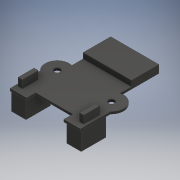
# Autodesk Inventor part: Encoder
Saved by Autodesk Inventor 2017 (Build 210142000, 142)
## iProperties
Part Number: Encoder
Material: Plástico ABS
Document SubType Name: Modeling
Designer: fam
Density: 1.06 g/cm^3
Appearance: Suave - Negro
Author: fam
Autodesk Inventor part; units mm, degrees
ref_plane "YZ Plane" through (0, 0, 0) normal (1, 0, 0) x (0, 1, 0)
ref_plane "XZ Plane" through (0, 0, 0) normal (0, 1, 0) x (-1, 0, 0)
ref_plane "XY Plane" through (0, 0, 0) normal (0, 0, 1) x (1, 0, 0)
sketch "Boceto1" plane through (0, 0, 0) normal (0, 0, 1) x (1, 0, 0)
  line L0 (-8, 26.74) -> (8, 26.74)
  line L1 (8, 26.74) -> (8, 0)
  line L2 (8, 0) -> (-8, 0)
  line L3 (-8, 0) -> (-8, 26.74)
  line L4 (6.17, 7.0485) -> (11.67, 7.0485)
  line L5 (11.67, 7.0485) -> (11.67, -3)
  line L6 (11.67, -3) -> (6.17, -3)
  line L7 (6.17, -3) -> (6.17, 7.0485)
  line L8 (-11.67, 7.0485) -> (-6.17, 7.0485)
  line L9 (-6.17, 7.0485) -> (-6.17, -3)
  line L10 (-6.17, -3) -> (-11.67, -3)
  line L11 (-11.67, -3) -> (-11.67, 7.0485)
  circle A0 centre (-9, 10) radius 1
  circle A1 centre (9, 10) radius 1
  circle A2 centre (-9, 10) radius 3.98
  circle A3 centre (9, 10) radius 3.98
  point P0 (0, 0)
  point P1 (0, 0)
  dimension "d0" = 16
  dimension "d1" = 26.74
  dimension "d2" = 5.5
  dimension "d3" = 23.34
  dimension "d6" = 11.67
  dimension "d7" = 29.74
  dimension "d8" = 2
  dimension "d9" = 25.96
  dimension "d10" = 13
  constraints: 24 end point, 6 horizontal, 6 vertical, 3 centre point, 3 horizontal alignment, 2 tangent, 1 coincident, 1 collinear, 1 concentric, 1 equal radius, 1 midpoint, 5 other
  measures "d0" distance of L1.end L2.end
  measures "d1" distance of L0.end L1.end
  measures "d2" distance of L5.end L6.end
  measures "d3" distance between parallel lines of L11 L5
  measures "d6" distance from line of point (0, 0) L5
  measures "d7" distance between parallel lines of L6 L0
  measures "d8" diameter of A1
  measures "d10" distance from line of L6 point (9, 10)
extrude "Extrusión1" add sketch "Boceto1" along normal blind 0.74
sketch "Boceto2" plane through (0, 0, 0.74) normal (0, 0, 1) x (1, 0, 0)
  line L0 (-8, 26.74) -> (8, 26.74)
  line L1 (8, 26.74) -> (8, 17.62)
  line L2 (8, 17.62) -> (-8, 17.62)
  line L3 (-8, 17.62) -> (-8, 26.74)
  point P0 (0, 0)
  dimension "d13" = 9.12
  constraints: 8 end point, 2 coincident, 2 horizontal, 2 vertical
  measures "d13" distance of L0.end L1.end
extrude "Extrusión2" add sketch "Boceto2" along normal blind 1.82
sketch "Boceto3" plane through (0, 0, 0.74) normal (0, 0, 1) x (1, 0, 0)
  line L0 (9.5, 4.2) -> (10.88, 4.2)
  line L1 (10.88, 4.2) -> (10.88, -1.1)
  line L2 (10.88, -1.1) -> (9.5, -1.1)
  line L3 (9.5, -1.1) -> (9.5, 4.2)
  line L4 (-10.88, 4.2) -> (-9.5, 4.2)
  line L5 (-9.5, 4.2) -> (-9.5, -1.1)
  line L6 (-9.5, -1.1) -> (-10.88, -1.1)
  line L7 (-10.88, -1.1) -> (-10.88, 4.2)
  line L8 (-11.67, 7.0485) -> (-11.67, -3) projected
  line L9 (6.17, -3) -> (11.67, -3) projected
  point P0 (0, 0)
  dimension "d16" = 5.3
  dimension "d17" = 1.38
  dimension "d18" = 19
  dimension "d19" = 0.79
  dimension "d20" = 7.2
  constraints: 16 end point, 4 horizontal, 3 equal length, 2 horizontal alignment, 2 vertical, 1 point on line
  measures "d16" distance of L6.end L4.start
  measures "d17" distance of L4.start L4.end
  measures "d18" distance between parallel lines of L3 L5
  measures "d19" distance between parallel lines of L8 L7
  measures "d20" distance between parallel lines of L9 L0
extrude "Extrusión3" add sketch "Boceto3" along normal blind 2.63
sketch "Boceto4" plane through (0, 0, 0) normal (0, 0, -1) x (-1, 0, 0)
  line L0 (-6.78, -2.6) -> (-11.54, -2.6)
  line L1 (-11.54, -2.6) -> (-11.54, 5.54)
  line L2 (-11.54, 5.54) -> (-6.78, 5.54)
  line L3 (-6.78, 5.54) -> (-6.78, -2.6)
  line L4 (11.54, -2.6) -> (6.78, -2.6)
  line L5 (6.78, -2.6) -> (6.78, 5.54)
  line L6 (6.78, 5.54) -> (11.54, 5.54)
  line L7 (11.54, 5.54) -> (11.54, -2.6)
  line L8 (8, 26.74) -> (-8, 26.74) projected
  point P0 (0, 0)
  dimension "d23" = 4.76
  dimension "d24" = 23.08
  dimension "d25" = 29.34
  dimension "d26" = 11.54
  dimension "d27" = 8.14
  constraints: 16 end point, 4 horizontal, 3 vertical, 2 horizontal alignment, 1 collinear, 1 point on line
  measures "d23" distance of L4.start L4.end
  measures "d24" distance between parallel lines of L1 L7
  measures "d25" distance between parallel lines of L8 L0
  measures "d26" distance from line of point (0, 0) L1
  measures "d27" distance of L6.end L4.start
extrude "Extrusión4" add sketch "Boceto4" along normal blind 6.03
shell "Vaciado1" thickness 0.65 removed faces 2 at (8.3667, 0.1133, -6.03) at (-8.3667, 2.8267, -6.03)
equation "\"d26\" = 0.5 * d24"
